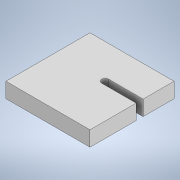
# Autodesk Inventor part: Support
Saved by Autodesk Inventor 2020 (Build 240168000, 168)
## iProperties
Created: 2019-11-07
Part Number: Support
Material: Générique
Document SubType Name: Modeling
Designer: erwan
Density: 1 g/cm^3
Appearance: Par défaut
Author: erwan
Autodesk Inventor part; units mm, degrees
ref_plane "YZ Plane" through (0, 0, 0) normal (1, 0, 0) x (0, 1, 0)
ref_plane "XZ Plane" through (0, 0, 0) normal (0, 1, 0) x (-1, 0, 0)
ref_plane "XY Plane" through (0, 0, 0) normal (0, 0, 1) x (1, 0, 0)
sketch "Esquisse1" plane through (0, 0, 0) normal (0, 1, 0) x (-1, 0, 0)
  line L0 (0, 0) -> (122, 0)
  line L1 (122, 0) -> (122, -122)
  line L2 (122, -122) -> (0, -122)
  line L3 (0, -122) -> (0, -77)
  line L4 (0, -77) -> (50, -77)
  arc A0 (50, -77) -> (50, -67) centre (50, -72) ccw
  line L5 (50, -67) -> (0, -67)
  line L6 (0, 0) -> (0, -67)
  dimension "d0" = 122
  dimension "d1" = 122
  dimension "d2" = 45
  dimension "d3" = 50
  constraints: 14 end point, 2 perpendicular, 2 point on circle, 1 centre point, 1 horizontal, 1 parallel, 1 vertical
  measures "d0" distance of L1.end L2.end
  measures "d1" distance of L0.end L1.end
  measures "d2" distance of L2.end L3.end
  measures "d3" distance of L3.end L4.end
extrude "Extrusion1" add sketch "Esquisse1" along normal blind 22
